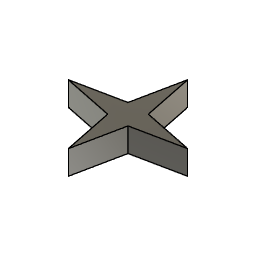
Homework1inProgress (Autodesk Fusion 360 design; units mm, degrees)
Autodesk Fusion 360 part; units mm, degrees
sketch "Sketch1" plane through (0, 0, 0) normal (0, 0, 1) x (1, 0, 0)
  line L0 (50, 0) -> (50, 50)
  line L1 (50, 50) -> (50, 100)
  line L2 (50, 50) -> (100, 50)
  line L3 (50, 50) -> (0, 50)
  line L4 (100, 50) -> (50, 60.2508)
  line L5 (50, 100) -> (60.2508, 50)
  line L6 (50, 100) -> (39.7492, 50)
  line L7 (0, 50) -> (50, 60.2508)
  line L8 (0, 50) -> (50, 39.7492)
  line L9 (50, 0) -> (39.7492, 50)
  line L10 (50, 0) -> (60.2508, 50)
  line L11 (100, 50) -> (50, 39.7492)
  constraint vertical L0
  constraint parallel L0 L1
  constraint perpendicular L1 L2
  constraint perpendicular L1 L3
  constraint coincident L1 L4.end
  constraint coincident L2 L5.end
  constraint coincident L3 L6.end
  constraint coincident L0 L8.end
extrude "Extrude1" add sketch "Sketch1" along normal blind 20
